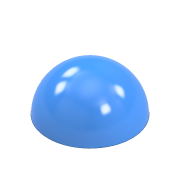
# Autodesk Inventor part: Ball
Saved by Autodesk Inventor 2020 (Build 240168000, 168)
## iProperties
Created: 2021-04-27
Part Number: Ball
Material: Generic
Document SubType Name: Modeling
Designer: deox
Density: 1 g/cm^3
Appearance: Cyan
Author: deox
Autodesk Inventor part; units mm, degrees
ref_plane "YZ Plane" through (0, 0, 0) normal (1, 0, 0) x (0, 1, 0)
ref_plane "XZ Plane" through (0, 0, 0) normal (0, 1, 0) x (-1, 0, 0)
ref_plane "XY Plane" through (0, 0, 0) normal (0, 0, 1) x (1, 0, 0)
sketch "Sketch1" plane through (0, 0, 0) normal (0, 0, 1) x (1, 0, 0)
  circle A0 centre (0, 0) radius 14.5044
  line L0 (0, 0) -> (0, 14.5044)
  line L1 (0, 0) -> (0, -14.5044)
  constraints: 4 end point, 2 point on circle, 2 vertical, 1 centre point, 1 coincident
revolve "Revolution1" add sketch "Sketch1" angle 360 about axis through (0, 0, 0) along (0, 1, 0) picked at (9.5484, -1.0758) contours A0 L1 L0
sketch "Sketch2" plane through (0, 0, 0) normal (0, 0, 1) x (1, 0, 0)
  line L0 (-17.5294, 0) -> (21.1361, 0)
  line L1 (21.1361, 0) -> (16.0945, -13.7482)
  line L2 (16.0945, -13.7482) -> (4.7314, -16.7344)
  line L3 (4.7314, -16.7344) -> (-11.3631, -14.9892)
  line L4 (-11.3631, -14.9892) -> (-16.6762, -5.2162)
  line L5 (-16.6762, -5.2162) -> (-19.512, 0)
  line L6 (-17.5294, 0) -> (-19.512, 0)
  point P0 (0, 0)
  constraints: 14 end point, 2 horizontal, 2 point on line
extrude "Extrusion1" cut sketch "Sketch2" against normal mid plane 30.5
body "Solid1"
